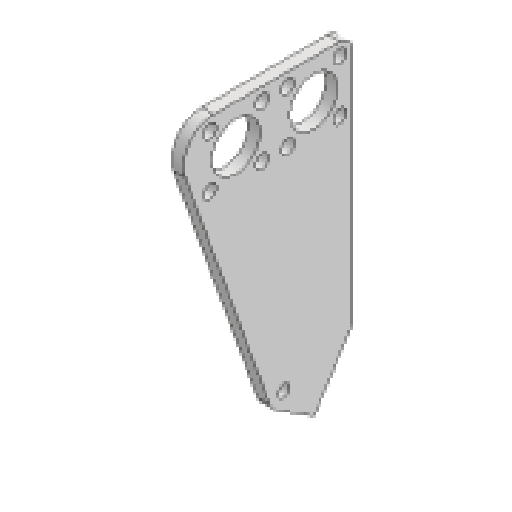
# Autodesk Inventor part: verticalSlidesPlate
Saved by Autodesk Inventor 2023 (Build 270158000, 158)
## iProperties
Created: 2022-10-26
Part Number: verticalSlidesPlate
Material: Generic
Document SubType Name: Modeling
Designer: deli
Density: 1 g/cm^3
Appearance: Default
Author: deli
Autodesk Inventor part; units mm, degrees
ref_plane "YZ Plane" through (0, 0, 0) normal (1, 0, 0) x (0, 1, 0)
ref_plane "XZ Plane" through (0, 0, 0) normal (0, 1, 0) x (-1, 0, 0)
ref_plane "XY Plane" through (0, 0, 0) normal (0, 0, 1) x (1, 0, 0)
sketch "Sketch1" plane through (0, 0, 0) normal (1, 0, 0) x (0, 1, 0)
  line L0 (480.2386, -480.8325) -> (469.5657, -497.7466) construction
  line L1 (469.5657, -497.7466) -> (215.8536, -337.6524) construction
  line L2 (215.8536, -337.6524) -> (226.5265, -320.7382) construction
  line L3 (226.5265, -320.7382) -> (480.2386, -480.8325) construction
  line L4 (226.5265, -320.7382) -> (-357.0113, 47.4786) construction
  line L5 (-357.0113, 47.4786) -> (-367.6843, 30.5644) construction
  line L6 (-367.6843, 30.5644) -> (215.8536, -337.6524) construction
  line L7 (-499.9626, 206.2365) -> (-499.9626, -867.2165) construction
  line L8 (-357.0113, 47.4786) -> (-360.817, 49.88) construction
  line L9 (-360.817, 49.88) -> (-371.4899, 32.9658) construction
  line L10 (-371.4899, 32.9658) -> (-367.6843, 30.5644) construction
  line L11 (-379.9626, 138.1186) -> (-379.9626, -322.1895) construction
  line L12 (-360.817, 49.88) -> (-369.6969, 55.4833) construction
  line L13 (-369.6969, 55.4833) -> (-367.9626, 58.2318) construction
  circle A0 centre (462.2165, -481.2848) radius 1.6
  circle A1 centre (348.0461, -409.2424) radius 1.6 construction
  circle A2 centre (233.8757, -337.2) radius 1.6 construction
  line L14 (350.9374, -635.582) -> (-499.9626, -635.582) construction
  line L15 (350.9374, -635.582) -> (350.9374, -660.982) construction
  line L16 (350.9374, -660.982) -> (-499.9626, -660.982) construction
  circle A3 centre (-53.3626, -140.2832) radius 4.25 construction
  line L17 (-451.9626, 107.1246) -> (-451.9626, -344.4416) construction
  line L18 (480.2386, -480.8325) -> (528.4439, -511.2504) construction
  circle A4 centre (530.7119, -507.6561) radius 4.25 construction
  line L19 (386.8939, -540.5479) -> (363.6374, -540.5479) construction
  line L20 (363.6374, -540.5479) -> (363.6374, -642.1479) construction
  line L21 (363.6374, -642.1479) -> (386.8939, -642.1479) construction
  line L22 (386.8939, -550.0729) -> (490.6374, -565.9479) construction
  line L23 (490.6374, -565.9479) -> (490.6374, -616.7479) construction
  line L24 (490.6374, -616.7479) -> (386.8939, -632.6229) construction
  line L25 (386.8939, -642.1479) -> (386.8939, -632.6229) construction
  line L26 (386.8939, -550.0729) -> (386.8939, -540.5479) construction
  line L27 (452.4299, -489.2987) -> (458.8337, -479.1503)
  arc A5 (460.8841, -477.5133) -> (458.8337, -479.1503) centre (462.2165, -481.2848) ccw
  line L28 (452.4299, -489.2987) -> (468.4984, -499.438)
  circle A6 centre (524.6749, -489.151) radius 6.35
  circle A7 centre (531.5897, -496.0658) radius 1.8288
  circle A8 centre (517.7601, -496.0658) radius 1.8288
  circle A9 centre (517.7601, -482.2362) radius 1.8288
  circle A10 centre (531.5897, -482.2362) radius 1.8288
  circle A11 centre (524.6749, -489.151) radius 7.9502 construction
  line L29 (531.5897, -482.2362) -> (531.5897, -496.0658) construction
  line L30 (531.5897, -496.0658) -> (517.7601, -496.0658) construction
  circle A12 centre (524.6749, -468.577) radius 6.35
  circle A13 centre (531.5897, -475.4918) radius 1.8288
  circle A14 centre (517.7601, -475.4918) radius 1.8288
  circle A15 centre (517.7601, -461.6622) radius 1.8288
  circle A16 centre (531.5897, -461.6622) radius 1.8288
  circle A17 centre (524.6749, -468.577) radius 7.9502 construction
  line L31 (531.5897, -461.6622) -> (531.5897, -475.4918) construction
  line L32 (531.5897, -475.4918) -> (517.7601, -475.4918) construction
  line L33 (468.4984, -499.438) -> (531.5897, -499.438)
  line L34 (534.9619, -496.0658) -> (534.9619, -462.6537)
  line L35 (524.2971, -455.1106) -> (460.8841, -477.5133)
  arc A18 (534.9619, -462.6537) -> (524.2971, -455.1106) centre (526.9619, -462.6537) ccw
  arc A19 (531.5897, -499.438) -> (534.9619, -496.0658) centre (531.5897, -496.0658) ccw
  point P0 (0, 0)
  point P1 (-368.8297, 56.8575)
  dimension "d24" = 8.5
  dimension "d0" = 20
  dimension "d1" = 300
  dimension "d2" = 690
  dimension "d3" = 4.5
  dimension "d4" = 120
  dimension "d5" = 10.5
  dimension "d6" = 3.25
  dimension "d7" = 12
  dimension "d8" = 3.2
  dimension "d9" = 10
  dimension "d10" = 10
  dimension "d11" = 10
  dimension "d12" = 15
  dimension "d13" = 135
  dimension "d14" = 135
  dimension "d15" = 25.4
  dimension "d16" = 850.9
  dimension "d17" = 8.5
  dimension "d18" = 3.25
  dimension "d19" = 372
  dimension "d21" = 48
  dimension "d22" = 398.6
  dimension "d23" = 57
  dimension "d26" = 101.6
  dimension "d27" = 50.8
  dimension "d28" = 8.7
  dimension "d29" = 8.7
  dimension "d30" = 127
  dimension "d31" = 82.55
  dimension "d32" = 898.6745
  dimension "d33" = 12.7
  dimension "d34" = 44.3245
  dimension "d36" = 8
  dimension "d37" = 2
  dimension "d38" = 12.7
  dimension "d39" = 3.6576
  dimension "d40" = 19.558
  dimension "d41" = 19.558
  dimension "d42" = 6.037
  dimension "d43" = 12.7
  dimension "d44" = 3.6576
  dimension "d45" = 19.558
  dimension "d46" = 19.558
  dimension "d47" = 6.037
  dimension "d48" = 20.574
  dimension "d49" = 10.287
  dimension "d50" = 4
  dimension "d51" = 10.287
  dimension "d52" = 8
  constraints: 72 end point, 19 centre point, 15 perpendicular, 13 tangent, 8 equal radius, 6 point on circle, 6 vertical, 5 coincident, 5 parallel, 4 collinear, 4 point on line, 3 equal length, 3 horizontal, 1 concentric, 1 midpoint, 4 other
  measures "d0" distance of L0.start L0.end
  measures "d1" distance of L2.end L0.start
  measures "d2" distance of L2.end L4.end
  measures "d3" distance of L4.end L8.end
  measures "d4" distance between parallel lines of L11 L7
  measures "d5" distance of L8.end L12.end
  measures "d6" distance of L12.end L13.end
  measures "d7" distance from line of L11 L13.end
  measures "d8" diameter of A0
  measures "d9" distance from line of L3 A0.centre
  measures "d10" distance from line of L3 A1.centre
  measures "d11" distance from line of L3 A2.centre
  measures "d12" distance from line of L0 A0.centre
  measures "d13" distance of A0.centre A1.centre
  measures "d14" distance of A2.centre A1.centre
  measures "d15" distance of L14.start L15.end
  measures "d16" distance of L14.start L14.end
  measures "d17" diameter of A3
  measures "d18" distance from line of L4 A3.centre
  measures "d19" distance of point (-368.83, 56.858) A3.centre
  measures "d21" distance between parallel lines of L17 L7
  measures "d22" distance from line of L17 A3.centre
  measures "d23" distance of L0.start L18.end
  measures "d26" distance of L20.end L19.end
  measures "d27" distance of L22.end L23.end
  measures "d28" angle of L21 L24
  measures "d29" angle of L22 L19
  measures "d30" distance between parallel lines of L20 L23
  measures "d31" distance of L24.end L22.start
  measures "d32" horizontal distance of point (530.712, -507.656) L13.end
  measures "d33" distance between parallel lines of L20 L15
  measures "d36" diameter of A5
  measures "d37" distance between parallel lines of L28 L1
  measures "d38" diameter of A6
  measures "d39" diameter of A7
  measures "d40" distance of L30.end L29.start
  measures "d41" distance of A7.centre A9.centre
  measures "d42" horizontal distance of A6.centre point (530.712, -507.656)
  measures "d43" diameter of A12
  measures "d44" diameter of A13
  measures "d45" distance of L32.end L31.start
  measures "d46" distance of A13.centre A15.centre
  measures "d47" horizontal distance of point (530.712, -507.656) A12.centre
  measures "d48" distance of A6.centre A12.centre
  measures "d49" distance from line of L33 A6.centre
  measures "d50" distance from line of A15.centre L35
  measures "d51" distance from line of L34 A11.centre
  measures "d52" radius of A18
extrude "Extrusion1" add sketch "Sketch1" along normal blind 3.175
sketch "Sketch2" plane through (0, 0, 0) normal (-1, 0, 0) x (0, 0, 1)
  line L0 (-499.438, 468.4984) -> (-499.438, 531.5897) projected
  line L1 (-499.438, 468.4984) -> (-497.7466, 469.5657)
  line L2 (-497.7466, 469.5657) -> (-487.6073, 453.4972)
  line L3 (-479.1503, 458.8337) -> (-489.2987, 452.4299) projected
  line L4 (-489.2987, 452.4299) -> (-499.438, 468.4984) projected
  point P0 (0, 0)
  dimension "d55" = 2
  constraints: 4 end point, 2 perpendicular, 1 point on line
  measures "d55" distance between parallel lines of L2 L4
extrude "Extrusion2" add sketch "Sketch2" along normal blind 3.175
equation "\"d9\" = 0.5 * d0"
equation "\"d10\" = d9"
equation "\"d11\" = d10"
equation "\"d13\" = -d12 + 0.5 * d1"
equation "\"d14\" = d13"
equation "\"d18\" = d6"
equation "\"d29\" = d28"
body "Solid1"
